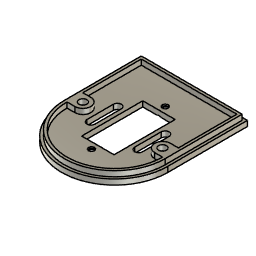
TRARM02_Link4A_30x40x2 (Autodesk Fusion 360 design; units mm, degrees)
Autodesk Fusion 360 part; units mm, degrees
note: some values were not read from the file. Set by a fixed rule: which sketch regions a step uses.
sketch "스케치1" plane through (0, 0, 0) normal (0, 0, 1) x (1, 0, 0)
  line L0 (20, 30) -> (20, 0)
  line L1 (-20, 30) -> (-20, 0)
  arc A0 (-20, 0) -> (20, 0) centre (0, 0) ccw
  line L2 (-20, 30) -> (20, 30)
  dimension "d1" = 40
  dimension "d128" = 30
  dimension "d129" = 20
  constraint coincident A0.centre origin
  constraint tangent L0 A0
  constraint vertical L0
  constraint parallel L0 L1
  constraint horizontal L0.start L1.start
  measures "d1" diameter of A0
  measures "d128" vertical distance of A0.centre L1.start
  measures "d129" distance of A0.centre L1
extrude "돌출1" add sketch "스케치1" along normal blind 2
sketch "스케치2" plane through (0, 0, 2) normal (0, 0, 1) x (-1, 0, 0)
  circle A0 centre (0, 8.75) radius 1.1
  circle A1 centre (0, -19.05) radius 1.1
  line L0 (6.1, -16.65) -> (-6.1, -16.65)
  line L1 (-6.1, -16.65) -> (-6.1, 6.35)
  line L2 (-6.1, 6.35) -> (6.1, 6.35)
  line L3 (6.1, 6.35) -> (6.1, -16.65)
  dimension "d7" = 2.2
  dimension "d8" = 27.8
  dimension "d9" = 8.75
  dimension "d11" = 23
  dimension "d12" = 2.4
  dimension "d13" = 12.2
  dimension "d14" = 6.1
  constraint equal A0 A1
  constraint horizontal L0
  constraint vertical L1
  constraint horizontal L2
  constraint vertical L3
  constraint vertical origin A0.centre
  constraint vertical origin A1.centre
  measures "d7" diameter of A0
  measures "d8" distance of A0.centre A1.centre
  measures "d9" distance of origin A0.centre
  measures "d11" distance of L0.end L1.end
  measures "d12" vertical distance of A1.centre L0.end
  measures "d13" distance of L0.start L0.end
  measures "d14" horizontal distance of origin L1.end
extrude "돌출2" cut sketch "스케치2" against normal blind 2
chamfer "챔퍼2" distance 1.5 angle 45 2 edges at (1.0256, 19.4478, 0) (1.0256, -8.3522, 0)
sketch "스케치14" plane through (0, 0, 2) normal (0, 0, 1) x (-1, 0, 0)
  line L0 (20, -30) -> (20, 0) construction
  line L1 (-20, 0) -> (-20, -30) construction
  arc A0 (20, 0) -> (-20, 0) centre (0, 0) ccw construction
  line L2 (19, -29) -> (19, 0)
  arc A1 (19, 0) -> (-19, 0) centre (0, 0) ccw
  line L3 (-19, 0) -> (-19, -29)
  line L4 (-15, -6) -> (-18, -6)
  line L5 (15, -6) -> (18, -6)
  line L6 (15, 0) -> (18, 0)
  arc A2 (15, 0) -> (15, -6) centre (15, -3) ccw
  line L7 (18, -28) -> (18, -6)
  line L8 (-18, -6) -> (-18, -28)
  line L9 (-15, 0) -> (-18, 0)
  arc A3 (18, 0) -> (-18, 0) centre (0, 0) ccw
  arc A4 (-15, -6) -> (-15, 0) centre (-15, -3) ccw
  line L10 (-20, -30) -> (20, -30)
  line L11 (18, -28) -> (-18, -28)
  line L12 (19, -29) -> (-19, -29)
  dimension "d112" = 3
  dimension "d113" = 3
  dimension "d120" = 3
  dimension "d121" = 1
  dimension "d124" = 6
  dimension "d125" = 6
  dimension "d126" = 3
  dimension "d130" = 1
  dimension "d131" = 1
  constraint coincident L6.end L7
  constraint perpendicular L6 L7
  constraint coincident L6 A2.start
  constraint horizontal L5
  constraint vertical L6.start A2.centre
  constraint coincident L6.start A2.start
  constraint horizontal L4
  constraint horizontal L9
  constraint vertical L8
  constraint equal L4 L9
  constraint vertical L4.end L9.end
  constraint coincident A0.centre L6
  constraint coincident A0.centre L9
  constraint concentric A0 A3
  constraint concentric A0 A1
  constraint tangent L2 A1
  constraint tangent A1 L3
  constraint vertical L7
  constraint horizontal L12
  constraint horizontal L11
  measures "d112" distance of L5.start L5.end
  measures "d113" distance of L4.start L4.end
  measures "d120" distance of L6.start L6.end
  measures "d121" distance of L3 L8
  measures "d124" distance of A0.centre L5
  measures "d125" distance of A0.centre L4
  measures "d126" radius of A4
  measures "d130" distance of L11 L12
  measures "d131" distance of L10 L12
extrude "돌출15" add sketch "스케치14" along normal blind 2
sketch "스케치16" plane through (0, 0, 4) normal (0, 0, 1) x (-1, 0, 0)
  circle A0 centre (-15, -3) radius 1.5
  circle A1 centre (15, -3) radius 1.5
  arc A2 (15, 0) -> (15, -6) centre (15, -3) ccw
  arc A3 (-15, -6) -> (-15, 0) centre (-15, -3) ccw
  dimension "d106" = 3
  constraint equal A0 A1
  constraint concentric A1 A2
  constraint concentric A0 A3
  measures "d106" diameter of A0
extrude "돌출17" cut sketch "스케치16" against normal blind 4
chamfer "챔퍼4" distance 2 angle 45 1 edges at (16.3985, 3.5424, 0)
chamfer "챔퍼4" distance 2 angle 45 1 edges at (-13.6015, 3.5424, 0)
sketch "스케치17" plane through (0, 0, 2) normal (0, 0, 1) x (-1, 0, 0)
  line L0 (7.5, 0) -> (7.5, -10)
  line L1 (10.5, 0) -> (10.5, -10)
  arc A0 (10.5, 0) -> (7.5, 0) centre (9, 0) ccw
  arc A1 (7.5, -10) -> (10.5, -10) centre (9, -10) ccw
  arc A2 (-7.5, 0) -> (-10.5, 0) centre (-9, 0) ccw
  line L2 (-10.5, 0) -> (-10.5, -10)
  line L3 (-7.5, 0) -> (-7.5, -10)
  arc A3 (-10.5, -10) -> (-7.5, -10) centre (-9, -10) ccw
  point P0 (6.1, -16.65)
  dimension "d133" = 3
  dimension "d134" = 10
  dimension "d136" = 3
  dimension "d137" = 10
  dimension "d139" = 9
  dimension "d140" = 9
  constraint vertical A0.centre A1.centre
  constraint equal A0 A1
  constraint tangent L0 A1
  constraint tangent L1 A1
  constraint tangent L1 A0
  constraint vertical A2.centre A3.centre
  constraint equal A2 A3
  constraint tangent L2 A3
  constraint tangent L3 A3
  constraint tangent A2 L3
  constraint horizontal A1.centre A3.centre
  constraint horizontal origin A0.centre
  constraint tangent A2 L2
  constraint tangent L0 A0
  measures "d133" diameter of A0
  measures "d134" distance of A0.centre A1.centre
  measures "d136" diameter of A2
  measures "d137" distance of A2.centre A3.centre
  measures "d139" distance of origin A0.centre
  measures "d140" distance of origin A2.centre
extrude "돌출18" cut sketch "스케치17" against normal blind 2
